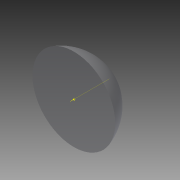
# Autodesk Inventor part: Comar39AF50
Saved by Autodesk Inventor 2015 SP1 (Build 190203100, 203)
## iProperties
Created: 2014-05-16
Part Number: Comar39AF50
Material: Glass
Document SubType Name: Modeling
Designer: ijs09
Density: 2.18 g/cm^3
Appearance: Clear - Blue
Author: ijs09
Autodesk Inventor part; units mm, degrees
ref_plane "YZ Plane" through (0, 0, 0) normal (1, 0, 0) x (0, 1, 0)
ref_plane "XZ Plane" through (0, 0, 0) normal (0, 1, 0) x (-1, 0, 0)
ref_plane "XY Plane" through (0, 0, 0) normal (0, 0, 1) x (1, 0, 0)
sketch "Sketch1" plane through (0, 0, 0) normal (0, 0, 1) x (1, 0, 0)
  line L0 (0, 0) -> (0, 19.5)
  line L1 (0, 0) -> (-25, 0)
  arc A0 (0, 19.5) -> (-25, 0) centre (1.8289, -8.6204) ccw
  dimension "d0" = 25
  dimension "d1" = 19.5
  constraints: 4 end point, 2 point on circle, 1 centre point, 1 perpendicular, 1 vertical
  measures "d0" distance of L0.start L1.end
  measures "d1" distance of L0.start L0.end
revolve "Revolution1" add sketch "Sketch1" angle 360 about axis through (0, 0, 0) along (0, 1, 0)
body "Solid1"
